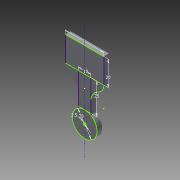
# Autodesk Inventor part: ToolHolder
Saved by Autodesk Inventor 2014 SP1 (Build 180222100, 222)
## iProperties
Created: 2014-07-12
Part Number: ToolHolder
Material: Generic
Document SubType Name: Modeling
Designer: Erin
Density: 1 g/cm^3
Appearance: Default
Author: Erin
Autodesk Inventor part; units mm, degrees
ref_plane "YZ Plane" through (0, 0, 0) normal (1, 0, 0) x (0, 1, 0)
ref_plane "XZ Plane" through (0, 0, 0) normal (0, 1, 0) x (-1, 0, 0)
ref_plane "XY Plane" through (0, 0, 0) normal (0, 0, 1) x (1, 0, 0)
sketch "Sketch1" plane through (0, 0, 0) normal (0, 1, 0) x (-1, 0, 0)
  line L0 (-5, 10.0042) -> (5, 10.0042)
  line L1 (5, 10.0042) -> (5, -14.9958)
  line L2 (5, -14.9958) -> (-5, -14.9958)
  line L3 (-5, -14.9958) -> (-5, 10.0042)
  circle A0 centre (0, -24.9958) radius 10
  circle A1 centre (0, -24.9958) radius 1.25
  line L4 (-5, -14.9958) -> (-5, -16.3355)
  line L5 (5, -14.9958) -> (5, -16.3355)
  line L6 (-15.5, 30.0042) -> (15.5, 30.0042)
  line L7 (15.5, 30.0042) -> (15.5, 10.0042)
  line L8 (15.5, 10.0042) -> (-15.5, 10.0042)
  line L9 (-15.5, 10.0042) -> (-15.5, 30.0042)
  arc A2 (-5, -5) -> (-10.4985, 2.7374) centre (-15.4294, -6.5891) ccw
  arc A3 (-15.5, 10.0042) -> (-10.4985, 2.7374) centre (-7.7202, 10.0042) ccw
  line L10 (0, 46.7954) -> (0, -49.019) construction
  line L11 (-15.5, 10.0042) -> (-5, 10.0042)
  point P0 (0, 0)
  point P1 (0, -14.9958)
  point P2 (0, 10.0042)
  point P3 (0, 10.0042)
  dimension "d0" = 25
  dimension "d1" = 10
  dimension "d2" = 20
  dimension "d3" = 2.5
  dimension "d6" = 31
  dimension "d7" = 20
  constraints: 24 end point, 6 parallel, 6 point on circle, 4 centre point, 3 midpoint, 2 coincident, 2 collinear, 2 horizontal, 2 perpendicular, 2 point on line, 2 tangent, 1 vertical, 1 vertical alignment
  measures "d0" distance of L2.end L0.start
  measures "d1" distance of L0.start L0.end
  measures "d2" diameter of A0
  measures "d3" diameter of A1
  measures "d6" distance of L6.start L6.end
  measures "d7" distance of L8.end L6.start
extrude "Extrusion1" add sketch "Sketch1" along normal blind 4.2 contours L8 L9 L6 L7 L0 | L0 L1 L2 L3 | L5 A0 L2 | L2 A0 L4 | A0
extrude "Extrusion2" add sketch "Sketch1" along normal blind 4.2 contours L3 A2 A3 L8
mirror "Mirror1" about plane through (0, 0, 0) normal (1, 0, 0) of "Extrusion2"
body "Solid1"
